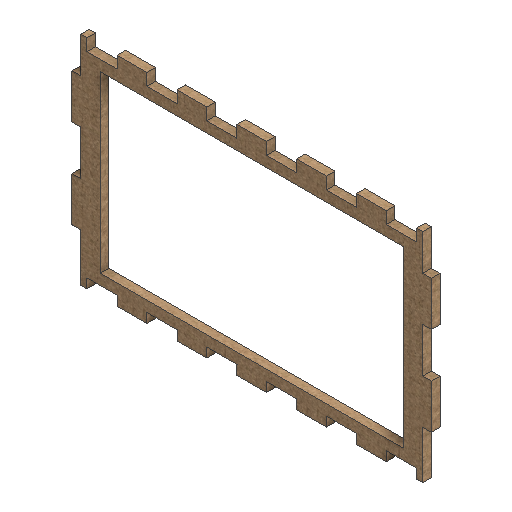
# Autodesk Inventor part: Frontplate
Saved by Autodesk Inventor 2025.2 (Build 292293000, 293)
## iProperties
Created: 2025-03-07
Part Number: Frontplate
Material: MDF Medium Density Fiberboard
Document SubType Name: Modeling
Designer: ahorat
Density: 0.8 g/cm^3
Appearance: Cardboard - Corrugated
Author: ahorat
Autodesk Inventor part; units mm, degrees
ref_plane "YZ Plane" through (0, 0, 0) normal (1, 0, 0) x (0, 1, 0)
ref_plane "XZ Plane" through (0, 0, 0) normal (0, 1, 0) x (-1, 0, 0)
ref_plane "XY Plane" through (0, 0, 0) normal (0, 0, 1) x (1, 0, 0)
sketch "Sketch1" plane through (0, 0, 0) normal (0, 0, 1) x (1, 0, 0)
  line L0 (-105, -65) -> (105, -65)
  line L1 (105, -65) -> (105, 65)
  line L2 (105, 65) -> (-105, 65)
  line L3 (-105, 65) -> (-105, -65)
  line L4 (-105, -65) -> (105, 65) construction
  line L5 (105, -65) -> (-105, 65) construction
  line L6 (-88.5, -51) -> (88.5, -51)
  line L7 (88.5, -51) -> (88.5, 51)
  line L8 (88.5, 51) -> (-88.5, 51)
  line L9 (-88.5, 51) -> (-88.5, -51)
  line L10 (-88.5, -51) -> (88.5, 51) construction
  line L11 (88.5, -51) -> (-88.5, 51) construction
  point P0 (0, 0)
  point P1 (-105, 0)
  dimension "d0" = 177
  dimension "d1" = 102
  dimension "d2" = 130
  dimension "d3" = 210
  constraints: 24 end point, 5 midpoint, 4 parallel, 2 horizontal, 2 perpendicular
  measures "d0" distance of L7.end L8.end
  measures "d1" distance of L6.end L7.end
  measures "d2" distance of L0.end L1.end
  measures "d3" distance from line of L1 point (-105, 0)
extrude "Extrusion1" add sketch "Sketch1" along normal blind 5 contours L3 L2 L1 L0 | L9 L8 L7 L6
sketch "Sketch2" plane through (0, 0, 5) normal (0, 0, 1) x (1, 0, 0)
  line L0 (-90, -50) -> (-80, -50) construction
  line L1 (-80, -50) -> (-80, 50)
  line L2 (-80, 50) -> (-90, 50) construction
  line L3 (-90, 50) -> (-90, -50)
  line L4 (-90, -50) -> (-80, 50) construction
  line L5 (-80, -50) -> (-90, 50) construction
  line L6 (-105, 65) -> (-105, -65) construction
  line L7 (-88.5, -51) -> (-88.5, 51) construction
  arc A0 (-80, 50) -> (-90, 50) centre (-85, 50) ccw
  arc A1 (-90, -50) -> (-80, -50) centre (-85, -50) ccw
  point P0 (0, 0)
  point P1 (-85, 0)
  dimension "d6" = 10
  dimension "d7" = 100
  dimension "d10" = 20
  constraints: 12 end point, 4 point on circle, 2 centre point, 2 midpoint, 2 parallel, 2 tangent, 1 horizontal, 1 horizontal alignment, 1 perpendicular
  measures "d6" distance of L1.end L2.end
  measures "d7" distance of L0.end L1.end
  measures "d10" distance from line of L6 point (-85, 0)
extrude "Extrusion2" [suppressed]
mirror "Mirror1" [suppressed]
sketch "Sketch3" plane through (0, 0, 0) normal (0, 0, -1) x (-1, 0, 0)
  line L0 (105, -65) -> (99.9, -65)
  line L1 (99.9, -65) -> (99.9, -38.95)
  line L2 (99.9, -38.95) -> (105, -38.95)
  line L3 (105, -38.95) -> (105, -65)
  line L4 (105, -13.05) -> (99.9, -13.05)
  line L5 (99.9, -13.05) -> (99.9, 13.05)
  line L6 (99.9, 13.05) -> (105, 13.05)
  line L7 (105, 13.05) -> (105, -13.05)
  line L8 (105, 65) -> (99.9, 65)
  line L9 (99.9, 65) -> (99.9, 38.95)
  line L10 (99.9, 38.95) -> (105, 38.95)
  line L11 (105, 38.95) -> (105, 65)
  line L12 (-105, -65) -> (-105, 65) projected
  line L13 (-105, 65) -> (-99.9, 65)
  line L14 (-99.9, 65) -> (-99.9, 38.95)
  line L15 (-99.9, 38.95) -> (-105, 38.95)
  line L16 (-105, 38.95) -> (-105, 65)
  line L17 (-105, 13.05) -> (-99.9, 13.05)
  line L18 (-99.9, 13.05) -> (-99.9, -13.05)
  line L19 (-99.9, -13.05) -> (-105, -13.05)
  line L20 (-105, -13.05) -> (-105, 13.05)
  line L21 (-105, -65) -> (-99.9, -65)
  line L22 (-99.9, -65) -> (-99.9, -38.95)
  line L23 (-99.9, -38.95) -> (-105, -38.95)
  line L24 (-105, -38.95) -> (-105, -65)
  line L25 (105, -65) -> (-105, -65) projected
  line L26 (-105, 65) -> (105, 65) projected
  point P0 (0, 0)
  point P1 (-105, 0)
  point P2 (-105, -13.05)
  dimension "d13" = 130
  dimension "d14" = 26.05
  dimension "d15" = 26.1
  dimension "d16" = 5.1
  constraints: 48 end point, 12 parallel, 9 point on line, 6 horizontal, 6 perpendicular, 2 collinear, 2 horizontal alignment, 2 midpoint
  measures "d13" distance between parallel lines of L25 L26
  measures "d14" distance of L0.end L1.end
  measures "d15" distance of L4.end L5.end
  measures "d16" distance between parallel lines of L3 L1
extrude "Extrusion3" cut sketch "Sketch3" against normal blind 10
sketch "Sketch4" plane through (-99.9, -65, 0) normal (0, -1, 0) x (1, 0, 0)
  line L0 (0, 5) -> (0, 0) projected
  line L1 (0, 0) -> (199.8, 0) projected
  line L2 (199.8, 0) -> (199.8, 5) projected
  line L3 (0, 5) -> (199.8, 5) projected
  point P0 (99.9, 0)
extrude "Extrusion4" add sketch "Sketch4" along normal blind 2
sketch "Sketch5" plane through (0, 0, 0) normal (0, 0, -1) x (-1, 0, 0)
  line L0 (99.9, 38.95) -> (99.9, 65) projected
  line L1 (-99.9, 65) -> (99.9, 65) projected
  line L2 (-99.9, 65) -> (-99.9, 38.95) projected
  line L3 (-99.9, 38.95) -> (-105, 38.95) projected
  line L4 (-105, 13.05) -> (-105, 38.95) projected
  line L5 (-105, 13.05) -> (-99.9, 13.05) projected
  line L6 (-99.9, 13.05) -> (-99.9, -13.05) projected
  line L7 (-99.9, -13.05) -> (-105, -13.05) projected
  line L8 (-105, -38.95) -> (-105, -13.05) projected
  line L9 (-105, -38.95) -> (-99.9, -38.95) projected
  line L10 (-99.9, -38.95) -> (-99.9, -67) projected
  line L11 (99.9, -67) -> (99.9, -38.95) projected
  line L12 (99.9, -38.95) -> (105, -38.95) projected
  line L13 (105, -13.05) -> (105, -38.95) projected
  line L14 (105, -13.05) -> (99.9, -13.05) projected
  line L15 (99.9, -13.05) -> (99.9, 13.05) projected
  line L16 (99.9, 13.05) -> (105, 13.05) projected
  line L17 (105, 38.95) -> (105, 13.05) projected
  line L18 (105, 38.95) -> (99.9, 38.95) projected
  line L19 (8.65, -67) -> (26.25, -67)
  line L20 (26.25, -67) -> (26.25, -61.4)
  line L21 (26.25, -61.4) -> (8.65, -61.4)
  line L22 (8.65, -61.4) -> (8.65, -67)
  line L23 (43.65, -61.4) -> (43.65, -67)
  line L24 (43.65, -67) -> (61.25, -67)
  line L25 (61.25, -61.4) -> (43.65, -61.4)
  line L26 (61.25, -67) -> (61.25, -61.4)
  line L27 (78.65, -61.4) -> (78.65, -67)
  line L28 (78.65, -67) -> (96.25, -67)
  line L29 (96.25, -61.4) -> (78.65, -61.4)
  line L30 (96.25, -67) -> (96.25, -61.4)
  line L31 (0, 0) -> (0, -124.7) construction
  line L32 (150.9327, -2.5) -> (-150.9327, -2.5) construction
  line L33 (-8.65, -67) -> (-26.25, -67)
  line L34 (-26.25, -67) -> (-26.25, -61.4)
  line L35 (-26.25, -61.4) -> (-8.65, -61.4)
  line L36 (-8.65, -61.4) -> (-8.65, -67)
  line L37 (-43.65, -61.4) -> (-43.65, -67)
  line L38 (-43.65, -67) -> (-61.25, -67)
  line L39 (-61.25, -61.4) -> (-43.65, -61.4)
  line L40 (-61.25, -67) -> (-61.25, -61.4)
  line L41 (-78.65, -61.4) -> (-78.65, -67)
  line L42 (-78.65, -67) -> (-96.25, -67)
  line L43 (-96.25, -61.4) -> (-78.65, -61.4)
  line L44 (-96.25, -67) -> (-96.25, -61.4)
  line L45 (99.9, -67) -> (-99.9, -67) projected
  line L46 (99.9, -67) -> (-99.9, -67) projected
  point P0 (17.45, -61.4)
  point P1 (52.45, -61.4)
  point P2 (87.45, -61.4)
  point P3 (0, -2.5)
  point P4 (-17.45, -61.4)
  point P5 (-52.45, -61.4)
  point P6 (-87.45, -61.4)
  dimension "d21" = 210
  dimension "d22" = 17.45
  dimension "d23" = 17.6
  dimension "d24" = 5.6
  dimension "d27" = 35
  constraints: 52 end point, 15 symmetric about line, 2 coincident, 2 horizontal, 2 midpoint, 2 parallel, 2 point on line, 1 perpendicular, 1 vertical
  measures "d21" distance between parallel lines of L8 L13
  measures "d22" horizontal distance of point (0, 0) point (17.45, -61.4)
  measures "d23" distance of L20.end L21.end
  measures "d24" distance of L19.end L20.end
  measures "d27" distance of L21.end L23.start
extrude "Extrusion5" cut sketch "Sketch5" against normal through all contours L28 L27 L29 L30 | L24 L23 L25 L26 | L44 L43 L41 L42 | L19 L22 L21 L20 | L40 L39 L37 L38 | L33 L34 L35 L36
sketch "Sketch7" plane through (0, 0, 0) normal (0, 0, -1) x (-1, 0, 0)
  line L0 (99.9, 53) -> (-99.9, 53) construction
  line L1 (8.65, 53) -> (26.25, 53)
  line L2 (26.25, 53) -> (26.25, 65)
  line L3 (26.25, 65) -> (8.65, 65)
  line L4 (8.65, 65) -> (8.65, 53)
  line L5 (43.65, 65) -> (43.65, 53)
  line L6 (43.65, 53) -> (61.25, 53)
  line L7 (61.25, 65) -> (43.65, 65)
  line L8 (61.25, 53) -> (61.25, 65)
  line L9 (78.65, 65) -> (78.65, 53)
  line L10 (78.65, 53) -> (96.25, 53)
  line L11 (96.25, 65) -> (78.65, 65)
  line L12 (96.25, 53) -> (96.25, 65)
  line L13 (99.9, 38.95) -> (99.9, 65) projected
  line L14 (-99.9, 65) -> (-99.9, 38.95) projected
  line L15 (-99.9, 65) -> (99.9, 65) projected
  line L16 (0, 0) -> (0, 28.7468) construction
  line L17 (-43.65, 65) -> (-43.65, 53)
  line L18 (-43.65, 53) -> (-61.25, 53)
  line L19 (-61.25, 65) -> (-43.65, 65)
  line L20 (-61.25, 53) -> (-61.25, 65)
  line L21 (-78.65, 65) -> (-78.65, 53)
  line L22 (-96.25, 65) -> (-78.65, 65)
  line L23 (-78.65, 53) -> (-96.25, 53)
  line L24 (-96.25, 53) -> (-96.25, 65)
  line L25 (-8.65, 53) -> (-26.25, 53)
  line L26 (-26.25, 53) -> (-26.25, 65)
  line L27 (-8.65, 65) -> (-8.65, 53)
  line L28 (-26.25, 65) -> (-8.65, 65)
  point P0 (0, 53)
  point P1 (17.45, 65)
  point P2 (52.45, 65)
  point P3 (87.45, 65)
  point P4 (-52.45, 65)
  point P5 (-87.45, 65)
  point P6 (-17.45, 65)
  dimension "d41" = 17.45
  dimension "d42" = 17.6
  dimension "d44" = 35
  dimension "d47" = 12
  constraints: 52 end point, 15 symmetric about line, 4 point on line, 3 horizontal, 2 midpoint, 2 parallel, 1 perpendicular, 1 vertical, 18 other
  measures "d41" horizontal distance of point (0, 53) point (17.45, 65)
  measures "d42" distance of L2.end L4.start
  measures "d44" distance of L4.start L5.start
  measures "d47" distance between parallel lines of L0 L15
extrude "Extrusion7" cut sketch "Sketch7" against normal blind 10
sketch "Sketch8" plane through (0, 0, 0) normal (0, 0, -1) x (-1, 0, 0)
  line L0 (26.25, 65) -> (26.25, 53) projected
  line L1 (26.25, 53) -> (8.65, 53) projected
  line L2 (8.65, 53) -> (8.65, 65) projected
  line L3 (-8.65, 65) -> (8.65, 65) projected
  line L4 (-8.65, 65) -> (-8.65, 53) projected
  line L5 (-8.65, 53) -> (-26.25, 53) projected
  line L6 (-26.25, 53) -> (-26.25, 65) projected
  line L7 (-43.65, 65) -> (-26.25, 65) projected
  line L8 (-43.65, 65) -> (-43.65, 53) projected
  line L9 (-43.65, 53) -> (-61.25, 53) projected
  line L10 (-61.25, 53) -> (-61.25, 65) projected
  line L11 (-78.65, 65) -> (-61.25, 65) projected
  line L12 (-78.65, 65) -> (-78.65, 53) projected
  line L13 (-78.65, 53) -> (-96.25, 53) projected
  line L14 (-96.25, 53) -> (-96.25, 65) projected
  line L15 (-99.9, 65) -> (-96.25, 65) projected
  line L16 (-99.9, 65) -> (-99.9, 38.95) projected
  line L17 (-99.9, 38.95) -> (-105, 38.95) projected
  line L18 (-105, 13.05) -> (-105, 38.95) projected
  line L19 (-105, 13.05) -> (-99.9, 13.05) projected
  line L20 (-99.9, 13.05) -> (-99.9, -13.05) projected
  line L21 (-99.9, -13.05) -> (-105, -13.05) projected
  line L22 (-105, -38.95) -> (-105, -13.05) projected
  line L23 (-105, -38.95) -> (-99.9, -38.95) projected
  line L24 (-99.9, -38.95) -> (-99.9, -67) projected
  line L25 (-96.25, -67) -> (-99.9, -67) projected
  line L26 (-96.25, -67) -> (-96.25, -61.4) projected
  line L27 (-96.25, -61.4) -> (-78.65, -61.4) projected
  line L28 (-78.65, -61.4) -> (-78.65, -67) projected
  line L29 (-61.25, -67) -> (-78.65, -67) projected
  line L30 (-61.25, -67) -> (-61.25, -61.4) projected
  line L31 (-61.25, -61.4) -> (-43.65, -61.4) projected
  line L32 (-43.65, -61.4) -> (-43.65, -67) projected
  line L33 (-26.25, -67) -> (-43.65, -67) projected
  line L34 (-26.25, -67) -> (-26.25, -61.4) projected
  line L35 (-26.25, -61.4) -> (-8.65, -61.4) projected
  line L36 (-8.65, -61.4) -> (-8.65, -67) projected
  line L37 (8.65, -67) -> (-8.65, -67) projected
  line L38 (8.65, -67) -> (8.65, -61.4) projected
  line L39 (8.65, -61.4) -> (26.25, -61.4) projected
  line L40 (26.25, -61.4) -> (26.25, -67) projected
  line L41 (43.65, -67) -> (26.25, -67) projected
  line L42 (43.65, -67) -> (43.65, -61.4) projected
  line L43 (43.65, -61.4) -> (61.25, -61.4) projected
  line L44 (61.25, -61.4) -> (61.25, -67) projected
  line L45 (78.65, -67) -> (61.25, -67) projected
  line L46 (78.65, -67) -> (78.65, -61.4) projected
  line L47 (78.65, -61.4) -> (96.25, -61.4) projected
  line L48 (96.25, -61.4) -> (96.25, -67) projected
  line L49 (99.9, -67) -> (96.25, -67) projected
  line L50 (99.9, -67) -> (99.9, -38.95) projected
  line L51 (99.9, -38.95) -> (105, -38.95) projected
  line L52 (105, -13.05) -> (105, -38.95) projected
  line L53 (105, -13.05) -> (99.9, -13.05) projected
  line L54 (99.9, -13.05) -> (99.9, 13.05) projected
  line L55 (99.9, 13.05) -> (105, 13.05) projected
  line L56 (105, 38.95) -> (105, 13.05) projected
  line L57 (105, 38.95) -> (99.9, 38.95) projected
  line L58 (99.9, 38.95) -> (99.9, 65) projected
  line L59 (96.25, 65) -> (99.9, 65) projected
  line L60 (96.25, 65) -> (96.25, 53) projected
  line L61 (96.25, 53) -> (78.65, 53) projected
  line L62 (78.65, 53) -> (78.65, 65) projected
  line L63 (61.25, 65) -> (78.65, 65) projected
  line L64 (61.25, 65) -> (61.25, 53) projected
  line L65 (61.25, 53) -> (43.65, 53) projected
  line L66 (43.65, 53) -> (43.65, 65) projected
  line L67 (26.25, 65) -> (43.65, 65) projected
  line L68 (99.9, 60) -> (-99.9, 60)
  point P0 (0, 0)
  point P1 (-99.9, -62)
  point P2 (99.9, -62)
  point P3 (-98.075, -67)
  point P4 (-98.075, 65)
  point P5 (-8.65, 60)
  point P6 (8.65, 60)
  point P7 (-43.65, 60)
  point P8 (-26.25, 60)
  point P9 (-78.65, 60)
  point P10 (-61.25, 60)
  point P11 (-96.25, 60)
  point P12 (96.25, 60)
  point P13 (61.25, 60)
  point P14 (78.65, 60)
  point P15 (26.25, 60)
  point P16 (43.65, 60)
  dimension "d53" = 5
  constraints: 4 point on line, 2 end point, 2 midpoint, 1 perpendicular
  measures "d53" distance from line of L68 point (-98.075, 65)
extrude "Extrusion8" cut sketch "Sketch8" against normal through all contours L67 L66 L68 L0 | L68 L4 L3 L2 | L64 L63 L62 L68 | L68 L8 L7 L6 | L60 L59 L58 L68 | L68 L12 L11 L10 | L68 L16 L15 L14
sketch "Sketch9" plane through (0, 0, 0) normal (0, 0, -1) x (-1, 0, 0)
  line L0 (88.5, -55.2) -> (-88.5, -55.2)
  line L1 (-88.5, -55.2) -> (-88.5, 46.8)
  line L2 (-88.5, 46.8) -> (88.5, 46.8)
  line L3 (88.5, 46.8) -> (88.5, -55.2)
  line L4 (88.5, -55.2) -> (-88.5, 46.8) construction
  line L5 (-88.5, -55.2) -> (88.5, 46.8) construction
  line L6 (-8.65, 60) -> (8.65, 60) projected
  line L7 (8.65, -67) -> (-8.65, -67) projected
  line L8 (8.65, 53) -> (26.25, 53) projected
  line L9 (17.45, 53) -> (-17.45, -61.4)
  line L10 (-8.65, -61.4) -> (-26.25, -61.4) projected
  point P0 (0, 0)
  point P1 (0, -4.2)
  dimension "d54" = 177
  dimension "d55" = 102
  constraints: 14 end point, 5 midpoint, 2 parallel, 1 horizontal, 1 perpendicular
  measures "d54" distance of L0.start L0.end
  measures "d55" distance of L0.end L1.end
extrude "Extrusion9" cut sketch "Sketch9" against normal blind 5
equation "\"d27\" = 0.166667 * d21"
equation "\"d44\" = 0.166667 * d46"
equation "\"d46\" = 210"
body "Solid1"
